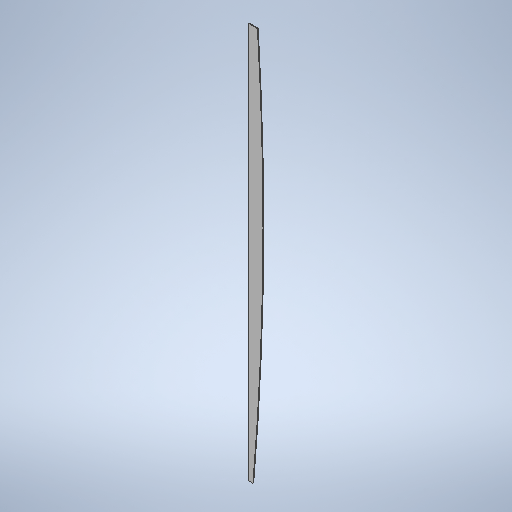
# Autodesk Inventor part: MSC 0512 rib back mould
Saved by Autodesk Inventor 2025 (Build 290162010, 162A)
## iProperties
Created: 2024-04-18
Part Number: MSC 0512 rib back mould
Material: AISI304
Document SubType Name: Sheet Metal
Designer: admin
Stock Number: МОО 024 лист борт основной
Mass: 48027.3 g
Surface Area: 40202.8 cm^2
Volume: 6003.41 cm^3
Density: 8 g/cm^3
Sheet Metal Rule: AISI304 3mm
Sheet Metal Width: 63,183 mm
Sheet Metal Length: 1700,000 mm
Sheet Metal Area: 107411,853 mm^2
Appearance: Default
Flat Pattern Width: 6.31834 cm
Flat Pattern Length: 170 cm
Flat Pattern Area: 1074.12 cm^2
Author: admin
Autodesk Inventor part; units mm, degrees
ref_plane "YZ Plane" through (0, 0, 0) normal (1, 0, 0) x (0, 1, 0)
ref_plane "XZ Plane" through (0, 0, 0) normal (0, 1, 0) x (-1, 0, 0)
ref_plane "XY Plane" through (0, 0, 0) normal (0, 0, 1) x (1, 0, 0)
sketch "Sketch1" plane through (0, 0, 0) normal (0, 0, 1) x (1, 0, 0)
  line L0 (-750, 0) -> (750, 0) construction
  line L1 (750, 0) -> (750, -2700) construction
  line L2 (750, -2700) -> (-750, -2700) construction
  line L3 (-750, -2700) -> (-750, 0) construction
  line L4 (800, 50) -> (-800, 50) construction
  line L5 (-800, 50) -> (-800, -2750) construction
  line L6 (-800, -2750) -> (800, -2750) construction
  line L7 (800, -2750) -> (800, 50) construction
  line L8 (-850, 100) -> (850, 100) construction
  line L9 (850, 100) -> (850, -2800) construction
  line L10 (850, -2800) -> (-850, -2800) construction
  line L11 (-850, -2800) -> (-850, 100) construction
  arc A0 (750, 0) -> (743.6915, 0.8413) centre (0, -5600) ccw construction
  line L12 (-750, -2100) -> (750, -2100) construction
  line L13 (115.486, -2697.8227) -> (669.21, -2176.1182) construction
  arc A1 (750, -2100) -> (750.1787, -2098.1258) centre (-10250, -1050) ccw construction
  line L14 (750, 0) -> (749.6018, -2.9735) construction
  arc A2 (750, -3.0268) -> (0, 47) centre (-0.2, -5603) ccw construction
  line L15 (750, 0) -> (747.0136, -0.2851) construction
  arc A3 (768.075, -251.105) -> (747.4657, -5.0326) centre (-10252.9897, -1050.251) ccw construction
  arc A4 (750.6027, -6.3335) -> (743.6915, 0.8413) centre (742.6385, -7.0891) ccw construction
  arc A5 (747.4657, -5.0326) -> (744.8748, -2.3426) centre (744.4792, -5.3164) ccw construction
  line L16 (750, -2100) -> (752.9864, -2100.2851) construction
  arc A6 (752.9864, -2100.2851) -> (772.2226, -225.7318) centre (-10246.9893, -1050.0309) ccw construction
  line L17 (750, -2100) -> (752.0572, -2102.1835) construction
  line L18 (752.0573, -2102.1835) -> (752.0572, -2102.1835) construction
  arc A7 (748.63, -2101.2908) -> (750.1787, -2098.1258) centre (745.2013, -2097.6516) ccw
  line L19 (0, -2697) -> (110.7938, -2697) construction
  line L20 (112.851, -2696.1835) -> (685.3487, -2156.791) construction
  arc A8 (110, -2700) -> (115.486, -2697.8227) centre (110, -2692) ccw construction
  arc A9 (110.7938, -2697) -> (112.851, -2696.1835) centre (110.7938, -2694) ccw construction
  line L21 (685.3487, -2156.791) -> (687.406, -2158.9745) construction
  line L22 (752.0573, -2102.1835) -> (671.2673, -2178.3017) construction
  line L23 (671.2673, -2178.3017) -> (669.21, -2176.1182) construction
  arc A10 (747.4657, -5.0326) -> (747.0136, -0.2851) centre (-10252.9897, -1050.251) ccw construction
  arc A11 (743.6915, 0.8413) -> (0, 50) centre (0, -5600) ccw construction
  arc A12 (750.6027, -6.3335) -> (750, 0) centre (-10250, -1050) ccw construction
  line L24 (771.0671, -250.888) -> (768.075, -251.105) construction
  line L25 (769.231, -225.9556) -> (772.2226, -225.7318) construction
  arc A13 (769.231, -225.9556) -> (750.6027, -6.3335) centre (-10250, -1050) ccw construction
  line L26 (0, 100) -> (0, 50) construction
  line L27 (0, -2700) -> (0, -2697) construction
  line L28 (0, 47) -> (0, 0) construction
  line L29 (0, 50) -> (0, 47) construction
  arc A14 (752.0572, -2102.1835) -> (752.9864, -2100.2851) centre (749.9998, -2099.9999) ccw construction
  line L30 (669.21, -2176.1182) -> (748.63, -2101.2908)
  arc A15 (750.1787, -2098.1258) -> (769.231, -225.9556) centre (-10250, -1050) ccw
  line L31 (748.63, -2101.2908) -> (750, -2100) construction
  line L32 (736.8166, -2025.9556) -> (756.8166, -2025.9556)
  line L33 (756.8166, -2025.9556) -> (756.8166, -325.9556) construction
  line L34 (756.8166, -325.9556) -> (736.8166, -325.9556)
  line L35 (736.8166, -325.9556) -> (736.8166, -2025.9556)
  line L36 (756.8166, -325.9556) -> (776.2532, -325.9556)
  line L37 (747.8166, -2025.9556) -> (747.8166, -2023.9556)
  line L38 (747.8166, -2023.9556) -> (745.8166, -2023.9556)
  line L39 (745.8166, -2023.9556) -> (745.8166, -2025.9556)
  point P0 (0, -2750)
  point P1 (749.6924, -2099.8492)
  point P2 (746.8166, -2023.9556)
  point P3 (746.8166, -2025.9556)
  dimension "d54" = 1500
  dimension "d55" = 2700
  dimension "d58" = 2100
  dimension "d68" = 8
  dimension "d70" = 3
  dimension "d75" = 5
  dimension "d83" = 8
  dimension "d86" = 3
  dimension "d112" = 251.771
  dimension "d113" = 50
  dimension "d114" = 50
  dimension "d115" = 3
  dimension "d116" = 25
  dimension "d117" = 110
  dimension "d118" = 25
  dimension "d119" = 111
  dimension "d121" = 1700
  dimension "d122" = 20
  dimension "d123" = 100
  dimension "d124" = 73.8937
  dimension "d125" = 150.1626
  dimension "d127" = 2
  measures "d54" distance of L0.start L0.end
  measures "d55" distance of L0.end L1.end
  measures "d58" distance between parallel lines of L12 L0
  measures "d68" radius of A4
  measures "d70" radius of A5
  measures "d75" radius of A7
  measures "d83" radius of A8
  measures "d86" radius of A9
  measures "d112" distance of L0.end L24.start
  measures "d113" distance between parallel lines of L4 L8
  measures "d114" distance between parallel lines of L0 L4
  measures "d115" distance of L26.end L28.start
  measures "d116" distance of L24.start L25.start
  measures "d117" distance from line of L27 A8.centre
  measures "d118" distance of L13.end L21.end
  measures "d119" distance of L12.end L13.end
  measures "d121" distance of L34.end L32.start
  measures "d122" distance of L32.start L32.end
  measures "d123" distance from line of L25.start L34
  measures "d124" vertical distance of L32.end point (749.692, -2099.849)
  measures "d125" vertical distance of L32.end L13.end
  measures "d127" distance of L38.end L39.end
extrude "Plate3" add sketch "Sketch1" along normal blind 3 contours L32 L37 L38 L39 L35 L34 L36 A15
equation "\"BendReliefWidth\" = Thickness"
equation "\"BendReliefDepth\" = 0.5 * Thickness"
equation "\"CornerReliefSize\" = 4 * Thickness"
equation "\"MinimumRemnant\" = 2 * Thickness"
equation "\"GapSize\" = Thickness"
equation "\"Thickness\" = 3"
body "Solid4"
